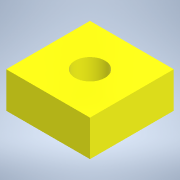
# Autodesk Inventor part: Soporte
Saved by Autodesk Inventor 2022 (Build 260153000, 153)
## iProperties
Created: 2022-01-26
Part Number: Soporte
Material: Genérico
Document SubType Name: Modeling
Designer: pc
Density: 1 g/cm^3
Appearance: Amarillo
Author: pc
Autodesk Inventor part; units mm, degrees
ref_plane "YZ Plane" through (0, 0, 0) normal (1, 0, 0) x (0, 1, 0)
ref_plane "XZ Plane" through (0, 0, 0) normal (0, 1, 0) x (-1, 0, 0)
ref_plane "XY Plane" through (0, 0, 0) normal (0, 0, 1) x (1, 0, 0)
sketch "Boceto1" plane through (0, 0, 0) normal (0, 1, 0) x (-1, 0, 0)
  line L0 (0, 0) -> (-1400, 0)
  line L1 (-1400, 0) -> (-1400, -1400)
  line L2 (-1400, -1400) -> (0, -1400)
  line L3 (0, -1400) -> (0, 0)
  dimension "d0" = 1400
  dimension "d1" = 1400
  constraints: 8 end point, 2 parallel, 1 horizontal, 1 perpendicular
  measures "d0" distance of L2.end L1.end
  measures "d1" distance of L1.end L0.end
extrude "Extrusión1" add sketch "Boceto1" along normal blind 600
sketch "Boceto2" plane through (0, 600, 0) normal (0, 1, 0) x (1, 0, 0)
  line L0 (0, 0) -> (800, 0)
  circle A0 centre (700, 700) radius 250
  line L1 (0, 1400) -> (0, 0) projected
  line L2 (1400, 1400) -> (0, 1400) projected
  dimension "d6" = 500
  dimension "d9" = 700
  dimension "d10" = 700
  constraints: 2 end point, 1 centre point, 1 horizontal
  measures "d6" diameter of A0
  measures "d9" distance from line of L1 A0.centre
  measures "d10" distance from line of L2 A0.centre
extrude "Extrusión2" cut sketch "Boceto2" against normal blind 400
